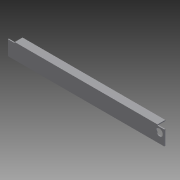
# Autodesk Inventor part: manipulator L frame left
Saved by Autodesk Inventor 2012 (Build 160160000, 160)
## iProperties
Created: 2013-09-01
Part Number: manipulator L frame left
Material: Default
Document SubType Name: Modeling
Designer: Bryce
Density: 1 g/cm^3
Author: Bryce
Autodesk Inventor part; units mm, degrees
ref_plane "YZ Plane" through (0, 0, 0) normal (1, 0, 0) x (0, 1, 0)
ref_plane "XZ Plane" through (0, 0, 0) normal (0, 1, 0) x (-1, 0, 0)
ref_plane "XY Plane" through (0, 0, 0) normal (0, 0, 1) x (1, 0, 0)
sketch "Sketch1" plane through (0, 0, 0) normal (0, 0, 1) x (1, 0, 0)
  line L0 (0, 0) -> (25.4, 0)
  line L1 (25.4, 0) -> (25.4, 3.175)
  line L2 (3.175, 50.8) -> (0, 50.8)
  line L3 (0, 50.8) -> (0, 0)
  line L4 (3.175, 50.8) -> (3.175, 3.175)
  line L5 (3.175, 3.175) -> (25.4, 3.175)
  dimension "d0" = 50.8
  dimension "d1" = 25.4
  dimension "d2" = 3.175
  dimension "d3" = 3.175
  constraints: 12 end point, 2 parallel, 1 horizontal, 1 perpendicular
  measures "d0" distance of L2.end L0.start
  measures "d1" distance of L0.start L0.end
  measures "d2" distance between parallel lines of L4 L3
  measures "d3" distance between parallel lines of L5 L0
extrude "Extrusion1" add sketch "Sketch1" along normal blind 508
sketch "Sketch2" plane through (0, 0, 0) normal (-1, 0, 0) x (0, 0, 1)
  line L0 (0, 0) -> (508, 0) projected
  line L1 (0, 50.8) -> (0, 0) projected
  circle A0 centre (15.875, 19.05) radius 11.1125
  dimension "d13" = 19.05
  dimension "d14" = 15.875
  dimension "d15" = 22.225
  constraints: 1 centre point
  measures "d13" distance from line of L0 A0.centre
  measures "d14" distance from line of L1 A0.centre
  measures "d15" diameter of A0
extrude "Extrusion2" cut sketch "Sketch2" against normal blind 508
sketch "Sketch3" plane through (0, 0, 0) normal (0, -1, 0) x (1, 0, 0)
  line L0 (25.4, 508) -> (0, 508) projected
  line L1 (0, 0) -> (0, 508) projected
  line L2 (25.4, 0) -> (25.4, 508) projected
  line L3 (0, 485.775) -> (25.4, 485.775)
  line L4 (0, 0) -> (25.4, 0) projected
  line L5 (0, 22.225) -> (25.4, 22.225)
  dimension "d16" = 22.225
  dimension "d19" = 22.225
  constraints: 4 end point, 4 point on line, 2 perpendicular
  measures "d16" distance between parallel lines of L0 L3
  measures "d19" distance between parallel lines of L4 L5
extrude "Extrusion3" cut sketch "Sketch3" against normal blind 3.175 contours L2 L3 L1 L0 | L2 L4 L1 L5
equation "\"d3\" = d2"
equation "\"d19\" = d16"
body "Solid1"
